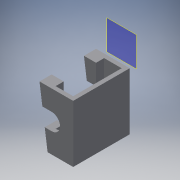
# Autodesk Inventor part: soporte baterias
Saved by Autodesk Inventor 2016 (Build 200138000, 138)
## iProperties
Created: 2017-02-23
Part Number: soporte baterias
Material: Generic
Document SubType Name: Modeling
Designer: jorge
Density: 1 g/cm^3
Appearance: Default
Author: jorge
Autodesk Inventor part; units mm, degrees
ref_plane "YZ Plane" through (0, 0, 0) normal (1, 0, 0) x (0, 1, 0)
ref_plane "XZ Plane" through (0, 0, 0) normal (0, 1, 0) x (-1, 0, 0)
ref_plane "XY Plane" through (0, 0, 0) normal (0, 0, 1) x (1, 0, 0)
sketch "Sketch1" plane through (0, 0, 0) normal (0, 0, 1) x (1, 0, 0)
  line L0 (-11.5, 1.5) -> (-11.5, 64) projected
  line L1 (-1.5, 1.5) -> (-11.5, 1.5) projected
  line L2 (-1.5, 64) -> (-1.5, 1.5) projected
  arc A0 (-1.5, 64) -> (-6, 68.5) centre (-6, 64) ccw projected
  line L3 (-7, 68.5) -> (-6, 68.5) projected
  arc A1 (-7, 68.5) -> (-11.5, 64) centre (-7, 64) ccw projected
  line L4 (-13, 64) -> (-13, 1.5) projected
  line L5 (0, 1.5) -> (0, 64) projected
  line L6 (-11.5, 0) -> (-1.5, 0) projected
  arc A2 (-13, 1.5) -> (-11.5, 0) centre (-11.5, 1.5) ccw projected
  arc A3 (-1.5, 0) -> (0, 1.5) centre (-1.5, 1.5) ccw projected
  arc A4 (-7, 70) -> (-13, 64) centre (-7, 64) ccw projected
  arc A5 (0, 64) -> (-6, 70) centre (-6, 64) ccw projected
  line L7 (-6, 70) -> (-7, 70) projected
  line L8 (-13, 1.5) -> (-13, 11.5)
  line L9 (-13, 64) -> (-13, 54)
  line L10 (0, 1.5) -> (0, 11.5)
  line L11 (0, 54) -> (0, 64)
  line L12 (0, 11.5) -> (3, 11.5)
  line L13 (3, 11.5) -> (3, 54)
  line L14 (3, 54) -> (0, 54)
  line L15 (0, 11.5) -> (0, 54)
  line L16 (-13, 11.5) -> (-16, 11.5)
  line L17 (-13, 54) -> (-22, 54)
  line L18 (-13, 11.5) -> (-13, 54)
  line L19 (-13, 11.5) -> (-13, 26.5)
  line L20 (-13, 26.5) -> (-18.1176, 26.5)
  line L21 (-13, 54) -> (-13, 39)
  line L22 (-13, 39) -> (-19.8824, 39)
  line L23 (-16, 11.5) -> (-18.1176, 26.5)
  line L24 (-19.8824, 39) -> (-22, 54)
  point P0 (0, 0)
  dimension "d0" = 10
  dimension "d1" = 10
  dimension "d2" = 3
  dimension "d3" = 3
  dimension "d4" = 9
  dimension "d5" = 15
  dimension "d6" = 15
  constraints: 34 end point, 7 point on line, 4 perpendicular, 3 horizontal, 2 parallel
  measures "d0" distance of L4.end L8.end
  measures "d1" distance of L4.start L9.end
  measures "d2" distance of L10.end L12.end
  measures "d3" distance of L8.end L16.end
  measures "d4" distance of L9.end L17.end
  measures "d5" distance of L8.end L19.end
  measures "d6" distance of L9.end L21.end
extrude "Extrusion1" add sketch "Sketch1" against normal blind 6 contours L4 L22 L24 L17 | L4 L16 L23 L20 | L14 L13 L12 L5
sketch "Sketch2" plane through (0, 0, 0) normal (0, 0, 1) x (1, 0, 0)
  line L0 (-18.1176, 26.5) -> (-16, 11.5) projected
  line L1 (-16, 11.5) -> (-13, 11.5) projected
  line L2 (-13, 26.5) -> (-18.1176, 26.5) projected
  line L3 (-19.8824, 39) -> (-13, 39) projected
  line L4 (-22, 54) -> (-19.8824, 39) projected
  line L5 (-13, 54) -> (-22, 54) projected
  line L6 (0, 11.5) -> (3, 11.5) projected
  line L7 (3, 11.5) -> (3, 54) projected
  line L8 (3, 54) -> (0, 54) projected
  line L9 (0, 11.5) -> (-13, 11.5)
  line L10 (-13, 54) -> (0, 54)
  arc A0 (-13, 26.5) -> (-13, 39) centre (-13, 32.75) ccw
  point P0 (0, 0)
  constraints: 4 end point, 2 point on circle, 2 tangent, 1 centre point, 1 horizontal, 1 parallel
extrude "Extrusion2" add sketch "Sketch2" along normal blind 3
ref_plane "Work Plane8" through (0, 70, -36) normal (0, 0, -1) x (-1, 0, 0)
sketch "Sketch3" plane through (0, 70, -36) normal (0, 0, -1) x (-1, 0, 0)
  line L0 (22, -16) -> (13, -16) projected
  line L1 (13, -16) -> (13, -31) projected
  line L2 (13, -31) -> (19.8824, -31) projected
  line L3 (19.8824, -31) -> (22, -16) projected
  line L4 (13, -43.5) -> (13, -58.5) projected
  line L5 (13, -58.5) -> (16, -58.5) projected
  line L6 (16, -58.5) -> (18.1176, -43.5) projected
  line L7 (18.1176, -43.5) -> (13, -43.5) projected
  line L8 (-3, -58.5) -> (0, -58.5) projected
  line L9 (0, -58.5) -> (0, -16) projected
  line L10 (0, -16) -> (-3, -16) projected
  line L11 (-3, -16) -> (-3, -58.5) projected
  point P0 (0, -70)
extrude "Extrusion3" add sketch "Sketch3" against normal blind 6
ref_plane "Work Plane7" through (0, 70, -36) normal (0, 0, -1) x (-1, 0, 0)
sketch "Sketch4" plane through (0, 70, -36) normal (0, 0, -1) x (-1, 0, 0)
  line L0 (22, -16) -> (13, -16) projected
  line L1 (13, -16) -> (13, -31) projected
  line L2 (13, -31) -> (19.8824, -31) projected
  line L3 (19.8824, -31) -> (22, -16) projected
  line L4 (13, -43.5) -> (13, -58.5) projected
  line L5 (13, -58.5) -> (16, -58.5) projected
  line L6 (16, -58.5) -> (18.1176, -43.5) projected
  line L7 (18.1176, -43.5) -> (13, -43.5) projected
  line L8 (-3, -58.5) -> (0, -58.5) projected
  line L9 (0, -58.5) -> (0, -16) projected
  line L10 (0, -16) -> (-3, -16) projected
  line L11 (-3, -16) -> (-3, -58.5) projected
  line L12 (18.1176, -43.5) -> (16, -58.5) projected
  line L13 (16, -58.5) -> (-3, -58.5) projected
  line L14 (-3, -58.5) -> (-3, -16) projected
  line L15 (-3, -16) -> (22, -16) projected
  line L16 (22, -16) -> (19.8824, -31) projected
  line L17 (19.8824, -31) -> (13, -31) projected
  arc A0 (13, -31) -> (13, -43.5) centre (13, -37.25) ccw projected
  line L18 (13, -43.5) -> (18.1176, -43.5) projected
  point P0 (0, -70)
extrude "Extrusion4" add sketch "Sketch4" along normal blind 3
sketch "Sketch5" plane through (0, 0, -6) normal (0, 0, -1) x (-1, 0, 0)
  line L0 (-3, 11.5) -> (0, 11.5) projected
  line L1 (0, 11.5) -> (0, 54) projected
  line L2 (0, 54) -> (-3, 54) projected
  line L3 (-3, 54) -> (-3, 11.5) projected
  point P0 (0, 0)
extrude "Extrusion5" add sketch "Sketch5" along normal up to next
body "Solid1"
